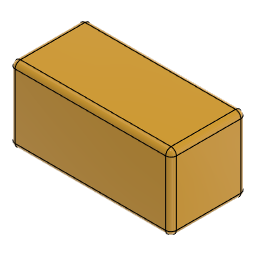
Assembly v2 (Autodesk Fusion 360 archive; units mm, degrees)
design "Battery"
Autodesk Fusion 360 part; units mm, degrees
sketch "Sketch1" plane through (0, 0, 0) normal (0, 0, 1) x (1, 0, 0)
  line L0 (0, 0) -> (75, 0)
  line L1 (75, 0) -> (75, 35)
  line L2 (75, 35) -> (0, 35)
  line L3 (0, 35) -> (0, 0)
  dimension "d1" = 75
  dimension "d2" = 35
  constraint horizontal L0
  constraint vertical L1
  constraint horizontal L2
  constraint vertical L3
  constraint coincident L0.start L3.end
  measures "d1" distance of L0.start L0.end
  measures "d2" distance of L0.start L2.end
extrude "Extrude1" add sketch "Sketch1" along normal blind 35
fillet "Fillet1" radius 2.5 12 edges at (37.5, 0, 35) (75, 0, 17.5) (75, 17.5, 35) (37.5, 35, 35) (0, 17.5, 35) (0, 35, 17.5) (37.5, 35, 0) (75, 35, 17.5) (75, 17.5, 0) (37.5, 0, 0) (0, 17.5, 0) (0, 0, 17.5)
